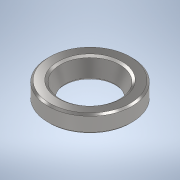
# Autodesk Inventor part: Кольцо поршень-шток верх
Saved by Autodesk Inventor 2021 (Build 250183000, 183)
## iProperties
Created: 2020-11-22
Part Number: Кольцо поршень-шток верх
Material: Сталь, мягкая
Document SubType Name: Modeling
Designer: Тимоха
Mass: 798.239 g
Surface Area: 194.798 cm^2
Volume: 101.686 cm^3
Density: 7.85 g/cm^3
Appearance: С умеренной полировкой
Author: Тимоха
Autodesk Inventor part; units mm, degrees
ref_plane "YZ Plane" through (0, 0, 0) normal (1, 0, 0) x (0, 1, 0)
ref_plane "XZ Plane" through (0, 0, 0) normal (0, 1, 0) x (-1, 0, 0)
ref_plane "XY Plane" through (0, 0, 0) normal (0, 0, 1) x (1, 0, 0)
sketch "Эскиз1" plane through (0, 0, 0) normal (0, 0, 1) x (1, 0, 0)
  line L0 (0, 0) -> (48.5, 0)
  line L1 (48.5, 0) -> (48.5, -20)
  line L2 (48.5, -20) -> (6.9412, -20)
  line L3 (0, 0) -> (35, 0)
  line L4 (35, 0) -> (27.7206, -20)
  line L5 (0, -24) -> (0, 4) projected
  dimension "d0" = 48.5
  dimension "d1" = 20
  dimension "d2" = 35
  dimension "d3" = 70
  constraints: 10 end point, 2 perpendicular, 1 horizontal, 1 midpoint, 1 point on line
  measures "d0" distance of L0.start L0.end
  measures "d1" distance of L0.end L1.end
  measures "d2" distance of L0.start L3.end
  measures "d3" angle of L0 L4
revolve "Вращение1" add sketch "Эскиз1" angle 360 about axis through (0, -10, 0) along (0, 1, 0)
chamfer "Фаска1" distance 2 angle 45 2 edges at (-35, 0, 0) (-27.7206, -20, 0)
chamfer "Фаска2" distance 2 angle 45 2 edges at (-48.5, -20, 0) (-48.5, 0, 0)
